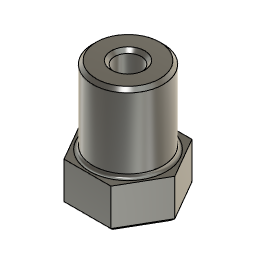
Gold flange replication v2 (Autodesk Fusion 360 design; units mm, degrees)
Autodesk Fusion 360 part; units mm, degrees
sketch "Sketch1" plane through (0, 0, 0) normal (0, 0, 1) x (1, 0, 0)
  line L0 (-5.5, 6) -> (-9, -0.0622)
  line L1 (-9, -0.0622) -> (-5.5, -6.1244)
  line L2 (-5.5, -6.1244) -> (1.5, -6.1244)
  line L3 (1.5, -6.1244) -> (5, -0.0622)
  line L4 (5, -0.0622) -> (1.5, 6)
  line L5 (1.5, 6) -> (-5.5, 6)
  point P0 (-2, -0.0622)
extrude "Extrude1" add sketch "Sketch1" along normal blind 6
sketch "Sketch2" plane through (0, 0, 6) normal (0, 0, 1) x (-1, 0, 0)
  line L0 (-1.5, -6) -> (5.5, -6)
  line L1 (5.5, -6) -> (9, 0.0622)
  line L2 (9, 0.0622) -> (5.5, 6.1244)
  line L3 (5.5, 6.1244) -> (-1.5, 6.1244)
  line L4 (-1.5, 6.1244) -> (-5, 0.0622)
  line L5 (-5, 0.0622) -> (-1.5, -6)
  circle A0 centre (2, 0.0622) radius 5.25
  dimension "d3" = 10.5
  measures "d3" diameter of A0
extrude "Extrude2" add sketch "Sketch2" along normal blind 11.5 contours A0
fillet "Fillet1" radius 0.5 1 edges at (2.8947, -1.9607, 6)
sketch "Sketch3" plane through (0, 0, 17.5) normal (0, 0, 1) x (-1, 0, 0)
  circle A0 centre (2, 0.0622) radius 5.25
  circle A1 centre (2, 0.0622) radius 2
  dimension "d8" = 4
  constraint concentric A0 A1
  measures "d8" diameter of A1
extrude "Extrude3" cut sketch "Sketch3" against normal blind 31.5 contours A1
chamfer "Chamfer1" distance 0.5 angle 45 2 edges at (-0.1353, -0.7854, 17.5) (2.8947, 1.8363, 17.5)
chamfer "Chamfer2" distance 0.5 angle 45 6 edges at (-2, -6.1244, 0) (-7.25, -3.0933, 0) (-7.25, 2.9689, 0) (-2, 6, 0) (3.25, 2.9689, 0) (3.25, -3.0933, 0)
